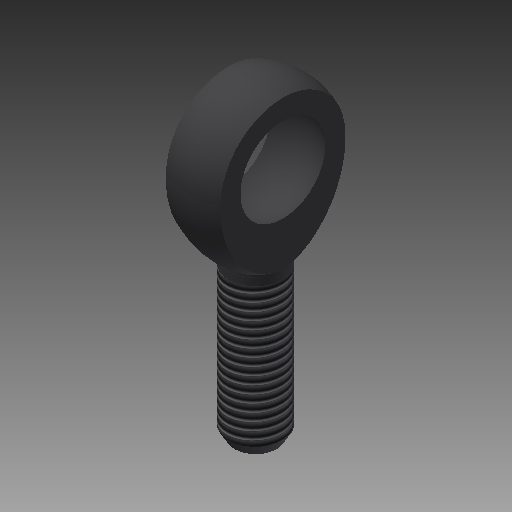
# Autodesk Inventor part: POS 12 Body
Saved by Autodesk Inventor 2018 (Build 220112000, 112)
## iProperties
Category: PARTsolutions
Company: IKO
Created: 2017-09-12
Part Number: POS 12 Body
Catalog Web Link: www.cadenas.de
Description: rod end with male thread BD-
Vendor: IKO
Document SubType Name: Modeling
Designer: psAdmin
Manufacturer: IKO
Mass: 9.16402 g
Surface Area: 42.5812 cm^2
Volume: 9.16402 cm^3
Density: 1 g/cm^3
Material: 一般
Appearance: PSOLRGB-128-128-128
PSOL_IDENT_0: {$CADENAS_DATA\23d-libs\iko\iko_bearings\pillobals\insert_type\rod_end_with_male_thread_body.prj},18
PSOL_IDENT_1: 5 {VTYP=3D},{NB=POS 12 Body},{LINA=POS 12 Body},{NN=rod end with male thread BD},{DATE=13.10.2016 10
PSOL_IDENT_2: :02:13},{GEOMDATE=03.12.2007 12:14:00},{VERSION=},{LINEID=70},{LINESUBID=-1},{WBVAR=}  {NB=POS 12 Bo
PSOL_IDENT_3: dy},{LINA=POS 12 Body},{KT=DUMMY},{IDNR=},{RID=G_70},{STDRT=12},{DESC=(gevmsg IKOSTV 914)},{TRNUMBER=
PSOL_IDENT_4: },{PAST=A},{REST=O},{ORDER=POS 12},{MASS=85.0},{SD=12},{G=M12x1.75},{NDM=12.000},{P1=1.750},{SD2=30}
PSOL_IDENT_5: ,{C1=12.0},{B=16},{SD1=15.4},{SL2=69},{SH=54},{SL1=33},{SR1=0.2},{DBL=22.23},{C2=0.00},{C3=0.00},{AA=
PSOL_IDENT_6: 0.00},{BB=0},{R2=3.0},{R3=22.5},{H2=41.03},{CGN=4.5},{P=2.5},{C=60},{LL6=34.56},{LL7=0.00},{LL8=2.34
PSOL_IDENT_7: },{LL9=0.00},{LL10=0.00},{CD=13100},{CS=16900},{G1=12},{GG1=10.11},{PP=1.8},{ALFA=55},{BL=4},{SC=1}
NN: rod end with male thread BD
NB: POS 12 Body
NBSYN: $ORDER. Body
LINA: POS 12 Body
RID: G_70
STDRT: 12
DESC: (gevmsg IKOSTV 914)
PAST: A
REST: O
ORDER: POS 12
MASS: 85.0
SD: 12
G: M12x1.75
NDM: 12.000
P1: 1.750
SD2: 30
C1: 12.0
B: 16
SD1: 15.4
SL2: 69
SH: 54
SL1: 33
SR1: 0.2
DBL: 22.23
C2: 0.00
C3: 0.00
AA: 0.00
BB: 0
R2: 3.0
R3: 22.5
H2: 41.03
CGN: 4.5
P: 2.5
C: 60
LL6: 34.56
LL7: 0.00
LL8: 2.34
LL9: 0.00
LL10: 0.00
CD: 13100
CS: 16900
G1: 12
GG1: 10.11
PP: 1.8
ALFA: 55
BL: 4
SC: 1
SUPPLIER: IKO
ARTICLENO: POS 12 Body
BOMINFO: POS 12 Body
CREATOR: CADENAS GmbH
Title: POS 12 Body
Author: Cadenas PARTsolutions
Autodesk Inventor part; units mm, degrees
sketch "Sketch_5" plane through (0, 0, 0) normal (0, 0, 1) x (1, 0, 0)
  line L0 (0, -33) -> (0, 36)
  arc A0 (15, 21) -> (0, 36) centre (0, 21) ccw
  arc A1 (6, 2.0892) -> (15, 21) centre (-7.4821, 20.1026) ccw
  arc A2 (6, 2.0892) -> (6, 1.56) centre (8.9883, 1.8246) ccw
  line L1 (6, 1.56) -> (6, -30.66)
  line L2 (6, -30.66) -> (4.649, -33)
  line L3 (4.649, -33) -> (0, -33)
  line L4 (0, -33) -> (0, 36)
  constraints: 10 end point, 6 point on circle, 3 centre point
revolve "Revolution1" add sketch "Sketch_5" angle 360 about axis through (0, -33, 0) along (0, -1, 0)
thread "Thread1" size "M12x1.75" class "6g" standard "ISO Metric profile" length 30.66
sketch "Sketch_6" plane through (0, 0, 0) normal (0, 0, 1) x (1, 0, 0)
  line L0 (-22.5, 37.8) -> (-22.5, -34.65)
  line L1 (-22.5, -34.65) -> (22.5, -34.65)
  line L2 (22.5, -34.65) -> (22.5, 37.8)
  line L3 (22.5, 37.8) -> (-22.5, 37.8)
  line L4 (-6, 36) -> (-6, -33)
  line L5 (-6, -33) -> (6, -33)
  line L6 (6, -33) -> (6, 36)
  line L7 (6, 36) -> (-6, 36)
  constraints: 16 end point
extrude "Extrusion1" cut sketch "Sketch_6" along normal mid plane 30
sketch "Sketch_7" plane through (0, 0, 0) normal (0, 0, 1) x (1, 0, 0)
  line L0 (11.115, 21) -> (-11.115, 21)
  arc A0 (11.115, 21) -> (-11.115, 21) centre (0, 21) ccw
  line L1 (11.115, 21) -> (-11.115, 21)
  constraints: 4 end point, 2 point on circle, 1 centre point
revolve "Revolution2" cut sketch "Sketch_7" angle 360 about axis through (11.115, 21, 0) along (1, 0, 0)
sketch "Sketch_14" plane through (0, 0, 0) normal (1, 0, 0) x (0, 1, 0)
  line L0 (6.5961, -13.8934) -> (10.1809, -8.7737)
  line L1 (10.1809, -8.7737) -> (12.024, -10.0643)
  line L2 (12.024, -10.0643) -> (8.4392, -15.184)
  line L3 (8.4392, -15.184) -> (6.5961, -13.8934)
  line L4 (6.5961, -13.8934) -> (10.1809, -8.7737)
  constraints: 10 end point
revolve "Revolution3" add sketch "Sketch_14" angle 360 about axis through (0, 6.5961, -13.8934) along (0, -0.5735764, -0.819152)
ref_plane "IP1_XY" through (0, 21, 0) normal (1, 0, 0) x (0, 0, -1)
ref_plane "IP1_YZ" through (0, 21, 0) normal (0, 0, -1) x (0, 1, 0)
ref_plane "IP1_ZX" through (0, 21, 0) normal (0, 1, 0) x (1, 0, 0)
body "Solid1"
